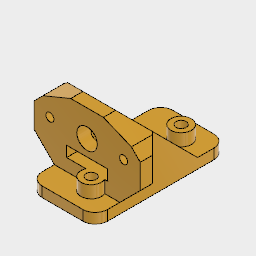
BLTouch_Bracket_v9 (Autodesk Fusion 360 design; units mm, degrees)
Autodesk Fusion 360 part; units mm, degrees
sketch "Sketch1" plane through (0, 0, 0) normal (0, 0, 1) x (1, 0, 0)
  circle A0 centre (0, 0) radius 1.25
  circle A1 centre (0, 22) radius 1.25
  line L0 (0, 0) -> (0, -5) construction
  line L1 (0, 0) -> (0, 1.25) construction
  line L2 (0, 20.75) -> (0, 22) construction
  line L3 (-7, 27) -> (3, 27)
  line L4 (6, 24) -> (6, -2)
  line L5 (3, -5) -> (-7, -5)
  line L6 (-10, -2) -> (-10, 24)
  arc A2 (-7, 27) -> (-10, 24) centre (-7, 24) ccw
  arc A3 (6, 24) -> (3, 27) centre (3, 24) ccw
  arc A4 (-10, -2) -> (-7, -5) centre (-7, -2) ccw
  arc A5 (3, -5) -> (6, -2) centre (3, -2) ccw
  circle A6 centre (0, 0) radius 2.5
  circle A7 centre (0, 22) radius 2.5
  line L7 (0, 22) -> (0, 27) construction
  dimension "d1" = 2.5
  dimension "d2" = 22
  dimension "d4" = 5
  dimension "d6" = 3
  dimension "d7" = 3
  dimension "d8" = 3
  dimension "d9" = 3
  dimension "d17" = 5
  dimension "d56" = 5
  constraint coincident A0
  constraint coincident A1
  constraint collinear L1 L2
  constraint horizontal L3
  constraint vertical L4
  constraint horizontal L5
  constraint tangent L3 A2
  constraint tangent L6 A2
  constraint tangent L3 A3
  constraint tangent L4 A3
  constraint tangent L5 A4
  constraint tangent L6 A4
  constraint tangent L4 A5
  constraint tangent L5 A5
  constraint concentric A1 A7
  constraint equal A6 A7
  constraint equal A0 A1
  constraint coincident L5
  constraint vertical L0
  constraint coincident L3
  constraint perpendicular L3 L7
  measures "d1" diameter of A0
  measures "d6" radius of A2
  measures "d7" radius of A3
  measures "d8" radius of A4
  measures "d9" radius of A5
  measures "d17" diameter of A6
extrude "Extrude1" add sketch "Sketch1" against normal blind 2.5 contours A0 | A1 | L3 L4 L5 L6 A2 A3 A4 A5 | A6 | A7
extrude "Extrude2" add sketch "Sketch1" along normal blind 3 contours A0 | A1 | A6 | A7
sketch "Sketch2" plane through (0, 0, 0) normal (0, 0, 1) x (1, 0, 0)
  arc A0 (-10, -2) -> (-7, -5) centre (-7, -2) ccw
  line L0 (-7, -5) -> (3, -5)
  arc A1 (3, -5) -> (6, -2) centre (3, -2) ccw
  line L1 (6, -2) -> (6, 24)
  arc A2 (6, 24) -> (3, 27) centre (3, 24) ccw
  line L2 (3, 27) -> (-7, 27)
  arc A3 (-7, 27) -> (-10, 24) centre (-7, 24) ccw
  line L3 (-10, 24) -> (-10, -2)
  circle A4 centre (0, 22) radius 2.5
  circle A5 centre (0, 0) radius 2.5
  line L4 (0, 0) -> (0, 1) construction
  line L5 (0, 1) -> (6, 1) construction
  line L6 (0, 1) -> (-10, 1) construction
  line L7 (-10, 1) -> (-7, 1)
  line L8 (-7, 1) -> (-7, 7)
  line L9 (-7, 7) -> (-10, 7)
  line L10 (-10, 7) -> (-10, 1)
  line L11 (6, 1) -> (3, 1)
  line L12 (3, 1) -> (3, 7)
  line L13 (3, 7) -> (6, 7)
  line L14 (6, 7) -> (6, 1)
  dimension "d60" = 1
  dimension "d61" = 3
  dimension "d62" = 6
  dimension "d63" = 6
  dimension "d64" = 3
  constraint coincident L1
  constraint perpendicular L1 L5
  constraint coincident L3
  constraint perpendicular L3 L6
  constraint horizontal L7
  constraint vertical L8
  constraint horizontal L9
  constraint vertical L10
  constraint horizontal L11
  constraint vertical L12
  constraint horizontal L13
  constraint vertical L14
extrude "Extrude3" add sketch "Sketch2" along normal blind 16 contours L3 L7 L8 L9 L10 | L1 L11 L12 L13 L14
chamfer "Chamfer1" distance 3 angle 45 2 edges at (-8.5, 7, 16) (4.5, 7, 16)
chamfer "Chamfer2" distance 13 angle 45 2 edges at (-8.5, 7, 0) (4.5, 7, 0)
sketch "Sketch3" plane through (-7, 0, 0) normal (1, 0, 0) x (0, 1, 0)
  line L0 (20, 0) -> (4, 16)
  line L1 (4, 16) -> (1, 16)
  line L2 (1, 16) -> (1, 0)
  line L3 (1, 16) -> (4, 16)
  line L4 (4, 16) -> (4, 0)
  line L5 (4, 0) -> (1, 0)
  line L6 (1, 0) -> (1, 16)
  constraint horizontal L3
  constraint vertical L4
  constraint horizontal L5
extrude "Extrude4" add sketch "Sketch3" along normal blind 18 and the other way blind 8
chamfer "Chamfer7" distance 5 angle 45 2 edges at (-15, 2.5, 16) (11, 2.5, 16)
chamfer "Chamfer3" distance 5 angle 45 2 edges at (-10, 4, 8) (6, 4, 8)
chamfer "Chamfer4" distance 3 angle 45 2 edges at (-7, 4, 8) (3, 4, 8)
sketch "Sketch4" plane through (0, 1, 0) normal (0, -1, 0) x (1, 0, 0)
  line L0 (-15, 16) -> (-15, 0)
  line L1 (-10, 0) -> (-2.5, 0)
  line L2 (-15, 0) -> (-10, 0)
  line L3 (11, 0) -> (11, 16)
  line L4 (11, 16) -> (-15, 16)
  circle A0 centre (-11.0787, 9.5) radius 1
  circle A1 centre (6.9213, 9.5) radius 1
  line L5 (-2.0787, 9.5) -> (6.9213, 9.5) construction
  line L6 (-2.0787, 9.5) -> (-11.0787, 9.5) construction
  line L7 (2.5, 0) -> (6, 0)
  line L8 (6, 0) -> (11, 0)
  line L9 (-2, 9.5) -> (-2, 16) construction
  line L10 (-7, 3) -> (3, 3)
  line L11 (3, 3) -> (3, 5.6)
  line L12 (3, 5.6) -> (-7, 5.6)
  line L13 (-7, 5.6) -> (-7, 3)
  circle A2 centre (-2, 9.5) radius 2.5
  line L14 (11, 11) -> (6, 16)
  line L15 (6, 16) -> (-10, 16)
  line L16 (-10, 16) -> (-15, 11)
  line L17 (-15, 11) -> (-15, 0)
  line L18 (-15, 0) -> (-10, 0)
  line L19 (-10, 0) -> (-2.2913, 0)
  line L20 (2.2913, 0) -> (6, 0)
  line L21 (6, 0) -> (11, 0)
  line L22 (11, 0) -> (11, 11)
  line L23 (-2, 9.5) -> (-2, 5.6) construction
  dimension "d39" = 2
  dimension "d45" = 9
  dimension "d46" = 9
  dimension "d48" = 6.5
  dimension "d51" = 10
  dimension "d52" = 2.6
  dimension "d55" = 5
  constraint equal A0 A1
  constraint coincident L6
  constraint midpoint L4
  constraint perpendicular L4 L9
  constraint horizontal L10
  constraint vertical L11
  constraint horizontal L12
  constraint vertical L13
  constraint horizontal L5
  constraint horizontal L6
  constraint midpoint L12
  constraint vertical L23
  measures "d39" diameter of A0
  measures "d55" diameter of A2
extrude "Extrude5" cut sketch "Sketch4" against normal blind 8 contours A0 | A1
chamfer "Chamfer8" distance 4 angle 45 2 edges at (6, 2.5, 16) (-10, 2.5, 16)
chamfer "Chamfer9" distance 5 angle 45 2 edges at (11, 2.5, 0) (-15, 2.5, 0)
extrude "Extrude6" cut sketch "Sketch4" against normal blind 6 contours L10 L11 L12 L13 | A2
extrude "Extrude7" cut sketch "Sketch1" along normal blind 3 and the other way blind 2.5 contours A0 | A1
